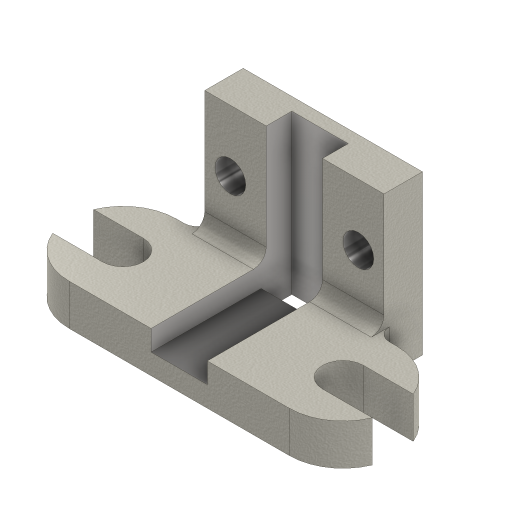
# Autodesk Inventor part: Part022. Corner piece
Saved by Autodesk Inventor 2023.2 (Build 272271030, 271C)
## iProperties
Created: 2023-09-21
Part Number: Part022. Corner piece
Material: Steel, Cast
Document SubType Name: Modeling
Designer: User
Mass: 862.247 g
Surface Area: 279.486 cm^2
Volume: 109.84 cm^3
Density: 7.85 g/cm^3
Appearance: Steel - Cast
Author: User
Autodesk Inventor part; units mm, degrees
ref_plane "YZ Plane" through (0, 0, 0) normal (1, 0, 0) x (0, 1, 0)
ref_plane "XZ Plane" through (0, 0, 0) normal (0, 1, 0) x (-1, 0, 0)
ref_plane "XY Plane" through (0, 0, 0) normal (0, 0, 1) x (1, 0, 0)
sketch "Sketch1" plane through (0, 0, 0) normal (0, 1, 0) x (-1, 0, 0)
  line L0 (43, 0) -> (-43, 0) construction
  line L1 (43, 21) -> (-43, 21)
  line L2 (-43, -21) -> (43, -21)
  arc A0 (43, -21) -> (43, 21) centre (43, 0) ccw
  arc A1 (-43, 21) -> (-43, -21) centre (-43, 0) ccw
  point P0 (0, 0)
  dimension "d0" = 43
  dimension "d1" = 21
  constraints: 8 end point, 4 point on circle, 4 tangent, 2 centre point, 1 horizontal, 1 midpoint, 1 parallel
  measures "d0" distance of point (0, 0) L0.end
  measures "d1" radius of A1
extrude "Extrusion1" add sketch "Sketch1" along normal blind 16
sketch "Sketch2" plane through (0, 16, 0) normal (0, 1, 0) x (1, 0, 0)
  arc A0 (43, -21) -> (43, 21) centre (43, 0) ccw projected
  arc A1 (-43, 21) -> (-43, -21) centre (-43, 0) ccw projected
  line L0 (-62.4165, 8) -> (-43, 8)
  arc A2 (-43, -8) -> (-43, 8) centre (-43, 0) ccw
  line L1 (-43, -8) -> (-62.4165, -8)
  line L2 (0, 29.4) -> (0, -29.4) construction
  line L3 (62.4165, 8) -> (43, 8)
  arc A3 (43, 8) -> (43, -8) centre (43, 0) ccw
  line L4 (43, -8) -> (62.4165, -8)
  point P0 (0, 0)
  dimension "d4" = 8
  constraints: 8 end point, 6 point on circle, 6 symmetric about line, 2 centre point, 2 coincident, 2 tangent, 1 horizontal, 1 parallel, 1 other
  measures "d4" radius of A2
extrude "Extrusion2" cut sketch "Sketch2" against normal through all
sketch "Sketch3" plane through (0, 0, 0) normal (0, 1, 0) x (-1, 0, 0)
  line L0 (35, -39) -> (-35, -39)
  line L1 (-35, -39) -> (-35, -24)
  line L2 (-35, -24) -> (35, -24)
  line L3 (35, -24) -> (35, -39)
  line L4 (43, 21) -> (-43, 21) projected
  point P0 (0, 0)
  point P1 (0, -24)
  point P2 (0, 21)
  dimension "d7" = 70
  dimension "d8" = 15
  dimension "d9" = 60
  constraints: 8 end point, 2 midpoint, 2 parallel, 1 horizontal, 1 perpendicular, 1 vertical alignment
  measures "d7" distance of L1.end L2.end
  measures "d8" distance of L0.end L1.end
  measures "d9" distance between parallel lines of L4 L0
extrude "Extrusion3" add sketch "Sketch3" along normal blind 62
sketch "Sketch4" plane through (0, 16, 0) normal (0, 1, 0) x (1, 0, 0)
  line L0 (43, 21) -> (-43, 21) projected
  line L1 (-35, 24) -> (35, 24) projected
  line L2 (-35, 24) -> (35, 24)
  line L3 (35, 24) -> (35, 21)
  line L4 (35, 21) -> (-35, 21)
  line L5 (-35, 21) -> (-35, 24)
  point P0 (0, 0)
  constraints: 8 end point, 2 parallel, 1 horizontal, 1 perpendicular, 1 point on line
extrude "Extrusion4" add sketch "Sketch4" against normal up to surface (16 mm away)
sketch "Sketch5" plane through (0, 62, 0) normal (0, 1, 0) x (1, 0, 0)
  line L0 (35, 39) -> (-35, 39) projected
  line L1 (-11, 34) -> (11, 34)
  line L2 (11, 34) -> (11, 22)
  line L3 (11, 22) -> (-11, 22)
  line L4 (-11, 22) -> (-11, 34)
  point P0 (0, 0)
  point P1 (0, 22)
  dimension "d14" = 5
  dimension "d15" = 22
  dimension "d16" = 12
  constraints: 8 end point, 2 parallel, 1 horizontal, 1 midpoint, 1 perpendicular, 1 vertical alignment
  measures "d14" distance between parallel lines of L0 L1
  measures "d15" distance of L1.start L1.end
  measures "d16" distance of L1.end L2.end
extrude "Extrusion5" cut sketch "Sketch5" against normal through all
sketch "Sketch6" plane through (-43, 0, 21) normal (0, 0, 1) x (1, 0, 0)
  line L0 (0, 0) -> (86, 0) projected
  line L1 (0, 16) -> (86, 16) projected
  line L2 (32, 16) -> (54, 16)
  line L3 (54, 16) -> (54, 8)
  line L4 (54, 8) -> (32, 8)
  line L5 (32, 8) -> (32, 16)
  line L6 (32, 16) -> (32, 62) projected
  line L7 (54, 62) -> (54, 16) projected
  point P0 (43, 0)
  dimension "d19" = 8
  constraints: 8 end point, 3 collinear, 2 parallel, 1 horizontal, 1 perpendicular
  measures "d19" distance between parallel lines of L0 L4
extrude "Extrusion6" cut sketch "Sketch6" against normal up to surface (55 mm away)
sketch "Sketch7" plane through (-11, 62, -24) normal (1, 0, 0) x (0, 0, -1)
  line L0 (0, -46) -> (0, 0) projected
  line L1 (-45, -46) -> (0, -46) projected
  arc A0 (-5, -46) -> (0, -41) centre (-5, -41) ccw
  point P0 (-24, -62)
  dimension "d22" = 5
  constraints: 2 point on circle, 2 point on line, 2 tangent, 1 centre point
  measures "d22" radius of A0
extrude "Extrusion7" add sketch "Sketch7" against normal up to surface (24 mm away)
mirror "Mirror1" about plane through (0, 0, 0) normal (1, 0, 0) of "Extrusion7"
fillet "Fillet1" radius 5 2 edges at (35, 8, -21) (-35, 8, -21)
sketch "Sketch8" plane through (-35, 62, -24) normal (0, 0, 1) x (1, 0, 0)
  line L0 (10, -24) -> (60, -24) construction
  line L1 (70, -62) -> (0, -62) projected
  point P0 (35, -62)
  point P1 (35, -24)
  dimension "d26" = 50
  dimension "d27" = 38
  constraints: 2 end point, 1 horizontal, 1 midpoint, 1 vertical alignment
  measures "d26" distance of L0.start L0.end
  measures "d27" distance between parallel lines of L1 L0
hole "Hole1" at (-25, 38, -24) at (25, 38, -24) direction (0, 0, -1) diameter 12 end through all
body "Solid1"
